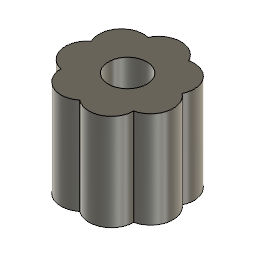
sugar macropad assembly (Autodesk Fusion 360 archive; units mm, degrees)
design "knob"
Autodesk Fusion 360 part; units mm, degrees
sketch "Sketch2" plane through (0, 0, 0) normal (0, 0, 1) x (1, 0, 0)
  circle A0 centre (0, 0) radius 8.5
  circle A1 centre (0, 0) radius 3
  circle A2 centre (0, 5) radius 3.5
  circle A3 centre (-3.9092, 3.1174) radius 3.5
  circle A4 centre (-4.8746, -1.1126) radius 3.5
  circle A5 centre (-2.1694, -4.5048) radius 3.5
  circle A6 centre (2.1694, -4.5048) radius 3.5
  circle A7 centre (4.8746, -1.1126) radius 3.5
  circle A8 centre (3.9092, 3.1174) radius 3.5
  dimension "d3" = 17
  dimension "d5" = 6
  dimension "d6" = 7
  dimension "d8" = 360
  constraint coincident A0.centre A1.centre
  constraint concentric A0 A1
  measures "d3" diameter of A0
  measures "d5" diameter of A1
  measures "d6" diameter of A2
extrude "Extrude1" add sketch "Sketch2" along normal blind 9 contours A1 A2 A7 A8 | A1 A2 A3 A8 | A1 A2 A8 | A1 A2 A3 A4 | A1 A2 A3 | A1 A7 A8 | A1 A6 A7 A8 | A1 A2 A3 A8 | A1 A2 A8 | A1 A3 A4 A5 | A1 A3 A4 | A1 A2 A3 A4 | A1 A2 A3 | A1 A2 A7 A8 | A1 A7 A8 | A1 A6 A7 A8 | A2 A3 A4 A5 A6 A7 A8 | A1 A4 A5 A6 | A1 A4 A5 | A1 A3 A4 A5 | A1 A3 A4 | A1 A6 A7 | A1 A6 A7 | A1 A5 A6 A7 | A1 A5 A6 | A1 A4 A5 A6 | A1 A4 A5 | A1 A5 A6 A7 | A1 A5 A6
extrude "Extrude2" add 1 faces at (1.3078, 0.2985, 9) along direction (0, 0, 1) blind 6
hole "Hole1" at (0.0633, 0.1229, 15) direction (0, 0, -1) diameter 6 depth 11 tip angle 180

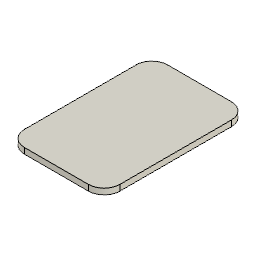
design "pad bottom"
part number: 2026-04-13-09-26-06-551
Autodesk Fusion 360 part; units mm, degrees
sketch "Sketch1" plane through (0, 0, 0) normal (0, 0, 1) x (1, 0, 0)
  line L0 (-48.3354, 60.7037) -> (-15.8354, 60.7037)
  line L1 (-7.8354, 52.7037) -> (-7.8354, -4.0463)
  line L2 (-15.8354, -12.0463) -> (-48.3354, -12.0463)
  line L3 (-56.3354, -4.0463) -> (-56.3354, 52.7037)
  arc A0 (-48.3354, 60.7037) -> (-56.3354, 52.7037) centre (-48.3354, 52.7037) ccw
  arc A1 (-7.8354, 52.7037) -> (-15.8354, 60.7037) centre (-15.8354, 52.7037) ccw
  arc A2 (-56.3354, -4.0463) -> (-48.3354, -12.0463) centre (-48.3354, -4.0463) ccw
  arc A3 (-15.8354, -12.0463) -> (-7.8354, -4.0463) centre (-15.8354, -4.0463) ccw
  point P0 (-56.3354, 60.7037)
  point P1 (-7.8354, 60.7037)
  point P2 (-56.3354, -12.0463)
  dimension "d1" = 48.5
  dimension "d2" = 72.75
  dimension "d3" = 8
  dimension "d4" = 8
  dimension "d5" = 8
  dimension "d6" = 8
  constraint horizontal L0
  constraint vertical L1
  constraint horizontal L2
  constraint vertical L3
  constraint coincident P0 L0
  constraint coincident P0 L3
  constraint tangent L0 A0
  constraint tangent L3 A0
  constraint coincident P1 L0
  constraint coincident P1 L1
  constraint tangent L0 A1
  constraint tangent L1 A1
  constraint coincident P2 L2
  constraint coincident P2 L3
  constraint tangent L2 A2
  constraint tangent L3 A2
  constraint tangent L1 A3
  constraint tangent L2 A3
  measures "d1" distance of P0 P1
  measures "d2" distance of P0 P2
  measures "d3" radius of A0
  measures "d4" radius of A1
  measures "d5" radius of A2
  measures "d6" radius of A3
extrude "Extrude1" add sketch "Sketch1" along normal blind 3
